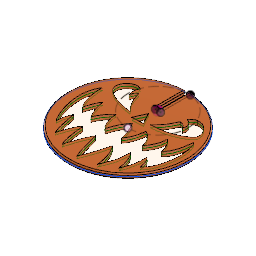
Halloween Disc Oloid (Autodesk Fusion 360 design; units mm, degrees)
Autodesk Fusion 360 part; units mm, degrees
sketch "Guides" plane through (0, 0, 0) normal (0, 0, 1) x (1, 0, 0)
  circle A0 centre (0, 0) radius 75 construction
  circle A1 centre (0, 0) radius 25 construction
  line L0 (-2.2, 0) -> (2.2, 0)
  line L1 (2.2, 0) -> (2.2, 24.9516)
  line L2 (-2.2, 24.9516) -> (-2.2, 0)
  arc A2 (-2.2, 24.9516) -> (2.2, 24.9516) centre (0, -25) ccw
  dimension "d1" = 150
  dimension "d2" = 50
  dimension "d3" = 4.4
  measures "d1" diameter of A0
  measures "d2" diameter of A1
sketch "Profile" plane through (0, 0, 0) normal (0, 0, 1) x (1, 0, 0)
  line L0 (-2.2, 0) -> (2.7, 0)
  line L1 (-2.2, 24.9516) -> (-2.2, 0)
  spline S0 degree 3 poles (-38.0449, -8.6936) (-48.1729, -24.3633) (-36.134, -48.4412) (-33.4587, -51.5942) knots 0 0 0 0 1 1 1 1
  spline S1 degree 2 poles (-33.4587, -51.5942) (-33.3631, -44.8104) (-30.5923, -39.8419) knots 0 0 0 1 1 1
  spline S2 degree 2 poles (-30.5923, -39.8419) (-27.2481, -57.0404) (-25.2416, -60.5756) knots 0 0 0 1 1 1
  spline S3 degree 3 poles (-25.2416, -60.5756) (-23.6173, -55.5116) (-20.8396, -46.1595) (-18.0756, -44.7148) knots 0 0 0 0 1 1 1 1
  spline S4 degree 3 poles (-18.0756, -44.7148) (-17.5979, -49.11) (-16.6424, -60.1934) (-13.776, -66.404) knots 0 0 0 0 1 1 1 1
  spline S5 degree 3 poles (-13.776, -66.404) (-11.8651, -59.0469) (-8.6165, -49.3966) (-5.9412, -46.3391) knots 0 0 0 0 1 1 1 1
  spline S6 degree 3 poles (-5.9412, -46.3391) (-4.3169, -52.1675) (-1.546, -63.7287) (0.9382, -68.6971) knots 0 0 0 0 1 1 1 1
  spline S7 degree 3 poles (0.9382, -68.6971) (3.0403, -63.3465) (6.0022, -55.5116) (8.1998, -46.0525) knots 0 0 0 0 1 1 1 1
  spline S8 degree 3 poles (8.1998, -46.0525) (10.8751, -49.3966) (14.1237, -54.2695) (15.5569, -66.1173) knots 0 0 0 0 1 1 1 1
  spline S9 degree 3 poles (15.5569, -66.1173) (20.7164, -53.6962) (20.5253, -50.7343) (20.812, -43.6638) knots 0 0 0 0 1 1 1 1
  spline S10 degree 3 poles (20.812, -43.6638) (24.5383, -46.9124) (26.2581, -53.6962) (27.2136, -59.9068) knots 0 0 0 0 1 1 1 1
  spline S11 degree 3 poles (27.2136, -59.9068) (31.131, -50.4476) (31.0355, -45.3837) (31.131, -40.1286) knots 0 0 0 0 1 1 1 1
  spline S12 degree 3 poles (31.131, -40.1286) (34.4752, -43.0905) (34.4752, -46.6258) (35.4306, -50.3521) knots 0 0 0 0 1 1 1 1
  spline S13 degree 3 poles (35.4306, -50.3521) (44.9853, -40.7019) (45.9408, -17.9617) (40.1124, -9.9358) knots 0 0 0 0 1 1 1 1
  spline S14 degree 3 poles (40.1124, -9.9358) (38.9659, -16.9107) (38.6792, -24.7455) (32.8509, -30.0006) knots 0 0 0 0 1 1 1 1
  spline S15 degree 3 poles (32.8509, -30.0006) (32.4687, -25.701) (29.9845, -21.4969) (26.7359, -18.6305) knots 0 0 0 0 1 1 1 1
  spline S16 degree 3 poles (26.7359, -18.6305) (26.4492, -21.0192) (26.8314, -25.8921) (20.7164, -33.8225) knots 0 0 0 0 1 1 1 1
  spline S17 degree 3 poles (20.7164, -33.8225) (20.0476, -30.0961) (16.9901, -23.9811) (12.0217, -21.8791) knots 0 0 0 0 1 1 1 1
  spline S18 degree 3 poles (12.0217, -21.8791) (11.3761, -24.3935) (11.2573, -31.5294) (6.3844, -36.7844) knots 0 0 0 0 1 1 1 1
  spline S19 degree 3 poles (6.3844, -36.7844) (5.62, -32.4848) (3.4224, -26.1787) (0.3649, -21.7836) knots 0 0 0 0 1 1 1 1
  spline S20 degree 3 poles (0.3649, -21.7836) (-2.6926, -25.701) (-5.4634, -30.5739) (-7.0877, -37.0711) knots 0 0 0 0 1 1 1 1
  spline S21 degree 3 poles (-7.0877, -37.0711) (-10.9096, -34.7779) (-12.3428, -27.6119) (-13.0116, -21.9747) knots 0 0 0 0 1 1 1 1
  spline S22 degree 3 poles (-13.0116, -21.9747) (-16.4513, -24.8411) (-20.3687, -31.0516) (-21.5153, -34.5869) knots 0 0 0 0 1 1 1 1
  spline S23 degree 3 poles (-21.5153, -34.5869) (-23.5218, -31.7204) (-26.1015, -26.5609) (-27.1526, -19.0127) knots 0 0 0 0 1 1 1 1
  spline S24 degree 3 poles (-27.1526, -19.0127) (-29.2871, -21.0727) (-30.3056, -24.65) (-32.2165, -30.765) knots 0 0 0 0 1 1 1 1
  spline S25 degree 3 poles (-32.2165, -30.765) (-34.8919, -28.3763) (-37.7583, -20.2548) (-38.0449, -8.6936) knots 0 0 0 0 1 1 1 1
  line L2 (0.1421, -7.9931) -> (-4.253, -17.7389)
  line L3 (-4.253, -17.7389) -> (5.1106, -17.2611)
  line L4 (5.1106, -17.2611) -> (0.1421, -7.9931)
  spline S26 degree 3 poles (-18.4414, 2.5358) (-20.2472, 2.3275) (-21.0322, 0.2572) (-21.8661, -2.3883) knots 0 0 0 0 1 1 1 1
  spline S27 degree 3 poles (-21.8661, -2.3883) (-23.4927, 1.4515) (-22.0912, 4.8343) (-21.1988, 6.4035) knots 0 0 0 0 1 1 1 1
  spline S28 degree 3 poles (-21.1988, 6.4035) (-21.4369, 6.5679) (-21.6827, 6.7257) (-21.9468, 6.8664) knots 0 0 0 0 1 1 1 1
  spline S29 degree 3 poles (-21.9468, 6.8664) (-28.6817, 10.4627) (-38.2387, -0.4036) (-31.0975, -6.5477) knots 0 0 0 0 1 1 1 1
  spline S30 degree 2 poles (-31.0975, -6.5477) (-24.5357, -12.193) (-9.2864, -13.9808) knots 0 0 0 1 1 1
  spline S31 degree 3 poles (-9.2864, -13.9808) (-14.8041, -9.0346) (-16.8748, -2.9058) (-18.4414, 2.5358) knots 0 0 0 0 1 1 1 1
  spline S32 degree 3 poles (25.605, 7.4412) (23.5461, 7.0769) (22.1859, 5.7259) (20.9912, 3.7477) knots 0 0 0 0 1 1 1 1
  spline S33 degree 3 poles (20.9912, 3.7477) (24.3621, 2.8633) (26.5631, -0.6062) (24.6098, -3.9282) knots 0 0 0 0 1 1 1 1
  spline S34 degree 3 poles (24.6098, -3.9282) (22.6067, -0.9524) (21.3467, -0.9089) (19.2603, -0.6532) knots 0 0 0 0 1 1 1 1
  spline S35 degree 3 poles (19.2603, -0.6532) (17.2286, -5.0904) (14.731, -10.1024) (9.1977, -15.3594) knots 0 0 0 0 1 1 1 1
  spline S36 degree 3 poles (9.1977, -15.3594) (21.8905, -14.9867) (32.4266, -9.6369) (36.2768, -5.9037) knots 0 0 0 0 1 1 1 1
  spline S37 degree 3 poles (36.2768, -5.9037) (40.0953, -2.0665) (33.5358, 8.8438) (25.605, 7.4412) knots 0 0 0 0 1 1 1 1
  line L5 (2.2, 0) -> (2.2, 24.9516)
  circle A0 centre (0, 0) radius 25 construction
  arc A1 (-2.2, 24.9516) -> (2.2, 24.9516) centre (0, -25) ccw
extrude "Extrude2" add sketch "Profile" along normal mid plane 4
chamfer "Chamfer1" distance 1 angle 45 2 edges at (0, -75, 2) (0, -75, -2)
extrude "Extrude1" [suppressed]
named bodies: "Halloween"
